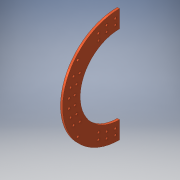
# Autodesk Inventor part: 13in inner coil
Saved by Autodesk Inventor 2016 (Build 200138000, 138)
## iProperties
Created: 2016-02-02
Part Number: 13in inner coil
Material: Copper
Document SubType Name: Modeling
Designer: Scott
Density: 8.94 g/cm^3
Appearance: Copper - Satin
Author: Scott
Autodesk Inventor part; units mm, degrees
ref_plane "YZ Plane" through (0, 0, 0) normal (1, 0, 0) x (0, 1, 0)
ref_plane "XZ Plane" through (0, 0, 0) normal (0, 1, 0) x (-1, 0, 0)
sketch "Sketch1" plane through (0, 0, 0) normal (1, 0, 0) x (0, 1, 0)
  arc A0 (165.1, 0) -> (-165.1, 0) centre (0, 0) ccw
  arc A1 (114.3, 0) -> (-114.3, 0) centre (0, 0) ccw
  line L0 (165.1, 0) -> (114.3, 0)
  line L1 (-114.3, 0) -> (-165.1, 0)
  circle A2 centre (0, 0) radius 130.81 construction
  circle A3 centre (0, 0) radius 147.32 construction
  line L2 (0, 0) -> (167.0124, 167.0124) construction
  line L3 (0, 0) -> (-143.9917, 143.9917) construction
  line L4 (0, 0) -> (0, 334.0248) construction
  point P0 (146.7716, 12.7)
  point P1 (142.4086, 37.7225)
  point P2 (130.192, 12.7)
  point P3 (125.2833, 37.6212)
  point P4 (133.8122, 61.6236)
  point P5 (115.6509, 61.1239)
  point P6 (12.7, 146.7716)
  point P7 (37.7225, 142.4086)
  point P8 (12.7, 130.192)
  point P9 (37.6212, 125.2833)
  point P10 (61.6236, 133.8122)
  point P11 (61.1239, 115.6509)
  point P12 (-146.7716, 12.7)
  point P13 (-142.4086, 37.7225)
  point P14 (-130.192, 12.7)
  point P15 (-125.2833, 37.6212)
  point P16 (-133.8122, 61.6236)
  point P17 (-115.6509, 61.1239)
  point P18 (-61.6236, 133.8122)
  point P19 (-37.7225, 142.4086)
  point P20 (-12.7, 146.7716)
  point P21 (-12.7, 130.192)
  point P22 (-37.6212, 125.2833)
  point P23 (-61.1239, 115.6509)
  dimension "d1" = 228.6
  dimension "d2" = 50.8
  dimension "d3" = 261.62
  dimension "d4" = 330.2
  dimension "d5" = 294.64
  dimension "d6" = 25.4
  dimension "d7" = 25.4
  dimension "d8" = 12.7
  dimension "d9" = 12.7
  dimension "d10" = 25.4
  dimension "d11" = 25.4
  dimension "d12" = 45
  dimension "d13" = 45
  constraints: 18 symmetric about line, 10 end point, 10 point on circle, 4 centre point, 4 coincident, 2 horizontal, 1 vertical
  measures "d1" diameter of A1
  measures "d2" distance of L0.start L0.end
  measures "d3" diameter of A2
  measures "d4" diameter of A0
  measures "d5" diameter of A3
  measures "d6" distance of A3.start A3.end
  measures "d7" distance of A2.start A2.end
  measures "d8" distance from line of L0 A2.start
  measures "d9" distance from line of L0 A3.start
  measures "d10" distance of A3.end point (133.812, 61.624)
  measures "d11" distance of A2.end point (115.651, 61.124)
  measures "d12" angle of L1 L3
  measures "d13" angle of L0 L2
extrude "Extrusion1" add sketch "Sketch1" along normal blind 6.35
hole "Hole1" at (0, 146.7716, 12.7) at (0, 142.4086, 37.7225) at (0, 130.192, 12.7) at (0, 125.2833, 37.6212) at (0, 133.8122, 61.6236) at (0, 115.6509, 61.1239) at (0, 61.6236, 133.8122) at (0, 37.7225, 142.4086) at (0, 12.7, 146.7716) at (0, 12.7, 130.192) at (0, 37.6212, 125.2833) at (0, 61.1239, 115.6509) at (0, -61.6236, 133.8122) at (0, -61.1239, 115.6509) at (0, -37.7225, 142.4086) at (0, -37.6212, 125.2833) at (0, -12.7, 146.7716) at (0, -12.7, 130.192) at (0, -115.6509, 61.1239) at (0, -133.8122, 61.6236) at (0, -142.4086, 37.7225) at (0, -125.2833, 37.6212) at (0, -146.7716, 12.7) at (0, -130.192, 12.7) direction (1, 0, 0) diameter 6.604 end through all
sketch "Sketch2" plane through (6.35, 0, 0) normal (1, 0, 0) x (0, 0, -1)
  circle A0 centre (-121.4655, -96.1901) radius 3.302 projected
  point P0 (0, 0)
extrude "Extrusion2" cut sketch "Sketch2" against normal blind 25.4
ref_plane "Work Plane1" through (6.35, 0, 177.8) normal (0, 1, 0) x (1, 0, 0)
mirror "Mirror1" about plane through (6.35, 0, 177.8) normal (0, 1, 0) of "Extrusion2"
body "Solid1"
